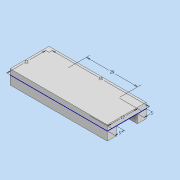
# Autodesk Inventor part: 모터 커버
Saved by Autodesk Inventor 2020 (Build 240168000, 168)
## iProperties
Created: 2020-05-07
Part Number: 모터 커버
Material: 일반
Document SubType Name: Modeling
Designer: sbahn
Density: 1 g/cm^3
Appearance: 기본값
Author: sbahn
Autodesk Inventor part; units mm, degrees
ref_plane "YZ Plane" through (0, 0, 0) normal (1, 0, 0) x (0, 1, 0)
ref_plane "XZ Plane" through (0, 0, 0) normal (0, 1, 0) x (-1, 0, 0)
ref_plane "XY Plane" through (0, 0, 0) normal (0, 0, 1) x (1, 0, 0)
sketch "스케치1" plane through (0, 0, 0) normal (0, 1, 0) x (-1, 0, 0)
  line L0 (0, 0) -> (55, 0)
  line L1 (55, 0) -> (55, -22)
  line L2 (55, -22) -> (0, -22)
  line L3 (0, -22) -> (0, 0)
  line L4 (55, -11) -> (0, -11) construction
  line L5 (27.5, 0) -> (27.5, -22) construction
  line L6 (42, -2.5) -> (13, -2.5)
  line L7 (13, -2.5) -> (13, -19.5)
  line L8 (13, -19.5) -> (42, -19.5)
  line L9 (42, -19.5) -> (42, -2.5)
  line L10 (42, -11) -> (13, -11) construction
  line L11 (27.5, -2.5) -> (27.5, -19.5) construction
  line L12 (55, -5) -> (0, -5)
  line L13 (0, -5) -> (0, -17)
  line L14 (0, -17) -> (55, -17)
  line L15 (55, -17) -> (55, -5)
  point P0 (27.5, -11)
  point P1 (27.5, -11)
  point P2 (0, -5)
  dimension "d0" = 55
  dimension "d1" = 22
  dimension "d2" = 29
  dimension "d3" = 17
  dimension "d4" = 5
  dimension "d5" = 5
  constraints: 32 end point, 10 midpoint, 6 parallel, 4 coincident, 3 horizontal, 3 perpendicular, 2 point on line
  measures "d0" distance of L1.end L2.end
  measures "d1" distance of L0.end L1.end
  measures "d2" distance of L8.end L7.end
  measures "d3" distance of L7.end L6.end
  measures "d4" distance between parallel lines of L2 L14
  measures "d5" distance between parallel lines of L0 L12
extrude "돌출1" add sketch "스케치1" along normal blind 3
extrude "돌출2" add sketch "스케치1" against normal blind 5 contours L0 L1 L12 L9 L6 L7 L3 | L14 L7 L8 L9 L1 L2 L3 | L7 L6 L9 L12 | L14 L9 L8 L7
